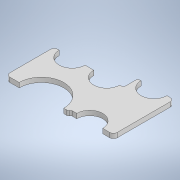
# Autodesk Inventor part: Top Bottle Middle
Saved by Autodesk Inventor 2021 (Build 250183000, 183)
## iProperties
Created: 2020-09-03
Part Number: Top Bottle Middle
Material: Generic
Document SubType Name: Modeling
Designer: jgray
Density: 1 g/cm^3
Appearance: Default
Author: jgray
Autodesk Inventor part; units mm, degrees
ref_plane "YZ Plane" through (0, 0, 0) normal (1, 0, 0) x (0, 1, 0)
ref_plane "XZ Plane" through (0, 0, 0) normal (0, 1, 0) x (-1, 0, 0)
ref_plane "XY Plane" through (0, 0, 0) normal (0, 0, 1) x (1, 0, 0)
sketch "Sketch1" plane through (0, 0, 0) normal (0, 1, 0) x (-1, 0, 0)
  circle A0 centre (18.5, 28) radius 23.85
  circle A1 centre (37, -23.25) radius 13.85
  circle A2 centre (-35, -38.75) radius 13.85
  circle A3 centre (-30.9, 25.8) radius 13.85
  circle A4 centre (0, -23.25) radius 13.85
  line L0 (56.25, 58.25) -> (-56.25, 58.25)
  line L1 (-56.25, -58.25) -> (56.25, -58.25)
  line L2 (0, -105.9299) -> (0, 123.2086) construction
  line L3 (-76.4777, -38.75) -> (-5.35, -38.75) construction
  line L4 (-123.5447, -23.25) -> (82.5572, -23.25) construction
  line L5 (56.25, -58.25) -> (56.25, 58.25)
  line L6 (56.25, 58.25) -> (56.25, -58.25)
  line L7 (-56.25, 58.25) -> (-56.25, -58.25)
  line L8 (100.0459, 28) -> (-13.85, 28) construction
  line L9 (-9.7154, 25.8) -> (-68.4996, 25.8) construction
  line L10 (18.5, 82.6038) -> (18.5, -4.654) construction
  line L11 (-30.9, 82.6038) -> (-30.9, 8.6393) construction
  point P0 (0, 0)
  point P1 (0, 0)
  dimension "d0" = 47.7
  dimension "d1" = 27.7
  dimension "d2" = 27.7
  dimension "d3" = 27.7
  dimension "d4" = 27.7
  dimension "d7" = 37
  dimension "d9" = 30.9
  dimension "d10" = 19.5
  dimension "d11" = 35
  dimension "d12" = 35
  dimension "d13" = 25.8
  dimension "d14" = 28
  dimension "d15" = 56.25
  dimension "d16" = 58.25
  dimension "d17" = 116.5
  dimension "d18" = 112.5
  dimension "d19" = 18.5
  dimension "d20" = 32.45
  constraints: 24 end point, 10 point on line, 5 centre point, 3 parallel, 2 horizontal, 2 perpendicular, 1 collinear, 1 vertical
  measures "d0" diameter of A0
  measures "d1" diameter of A1
  measures "d2" diameter of A2
  measures "d3" diameter of A3
  measures "d4" diameter of A4
  measures "d7" distance of A4.centre A1.centre
  measures "d9" distance from line of A3.centre L2
  measures "d10" distance between parallel lines of L1 L3
  measures "d11" distance between parallel lines of L1 L4
  measures "d12" horizontal distance of A2.centre A4.centre
  measures "d13" vertical distance of point (0, 0) A3.centre
  measures "d14" vertical distance of point (0, 0) A0.centre
  measures "d15" distance from line of point (0, 0) L5
  measures "d16" distance from line of L1 point (0, 0)
  measures "d17" distance between parallel lines of L1 L0
  measures "d18" distance between parallel lines of L7 L5
  measures "d19" horizontal distance of A0.centre point (0, 0)
  measures "d20" distance between parallel lines of L0 L9
extrude "Extrusion1" add sketch "Sketch1" along normal blind 5
sketch "Sketch2" plane through (0, 5, 0) normal (0, 1, 0) x (1, 0, 0)
  line L0 (-56.25, 58.25) -> (-56.25, -58.25) projected
  line L1 (-56.25, -58.25) -> (56.25, -58.25) projected
  line L2 (56.25, -58.25) -> (56.25, 58.25) projected
  line L3 (56.25, 58.25) -> (-56.25, 58.25) projected
  circle A0 centre (0, 23.25) radius 13.85 projected
  circle A1 centre (30.9, -25.8) radius 13.85 projected
  circle A2 centre (35, 38.75) radius 13.85 projected
  circle A3 centre (-37, 23.25) radius 13.85 projected
  circle A4 centre (-18.5, -28) radius 23.85 projected
  line L4 (-56.25, 58.25) -> (-56.25, -58.25) projected
  line L5 (-56.25, 23.25) -> (15.75, 23.25)
  line L6 (19.75, 38.75) -> (56.25, 38.75)
  line L7 (56.25, -58.25) -> (56.25, 58.25) projected
  line L8 (17.75, 25.25) -> (17.75, 36.75)
  arc A5 (15.75, 23.25) -> (17.75, 25.25) centre (15.75, 25.25) ccw
  arc A6 (19.75, 38.75) -> (17.75, 36.75) centre (19.75, 36.75) ccw
  point P0 (0, 0)
  point P1 (17.75, 23.25)
  point P2 (17.75, 38.75)
  point P3 (-50.85, 23.25)
  point P4 (-23.15, 23.25)
  point P5 (-13.85, 23.25)
  point P6 (13.85, 23.25)
  point P7 (21.15, 38.75)
  point P8 (48.85, 38.75)
  dimension "d23" = 74
  dimension "d25" = 38.5
  dimension "d26" = 2
  dimension "d27" = 35
  dimension "d28" = 19.5
  constraints: 6 end point, 6 point on line, 4 point on circle, 4 tangent, 2 centre point, 1 equal radius, 1 horizontal, 1 parallel, 1 vertical
  measures "d23" distance of point (17.75, 23.25) L5.start
  measures "d25" distance of point (17.75, 38.75) L6.end
  measures "d26" radius of A5
  measures "d27" distance between parallel lines of L3 L5
  measures "d28" distance between parallel lines of L3 L6
sketch "Sketch3" plane through (0, 5, 0) normal (0, 1, 0) x (1, 0, 0)
  line L0 (-56.25, -28) -> (8.75, -28)
  line L1 (12.3221, -25.8) -> (56.25, -25.8)
  line L2 (-56.25, 58.25) -> (-56.25, -58.25) projected
  line L3 (-56.25, -58.25) -> (56.25, -58.25) projected
  line L4 (56.25, -58.25) -> (56.25, 58.25) projected
  line L5 (56.25, 58.25) -> (-56.25, 58.25) projected
  circle A0 centre (0, 23.25) radius 13.85 projected
  circle A1 centre (30.9, -25.8) radius 13.85 projected
  circle A2 centre (35, 38.75) radius 13.85 projected
  circle A3 centre (-37, 23.25) radius 13.85 projected
  circle A4 centre (-18.5, -28) radius 23.85 projected
  line L6 (56.25, -58.25) -> (56.25, 58.25) projected
  line L7 (-56.25, 58.25) -> (-56.25, -58.25) projected
  line L8 (10.75, -26) -> (10.75, -25.8)
  arc A5 (8.75, -28) -> (10.5361, -26.9) centre (8.75, -26) ccw
  arc A6 (12.3221, -25.8) -> (10.5361, -26.9) centre (12.3221, -27.8) ccw
  point P0 (0, 0)
  point P1 (10.75, -28)
  point P2 (44.75, -25.8)
  point P3 (17.05, -25.8)
  point P4 (5.35, -28)
  point P5 (-42.35, -28)
  dimension "d29" = 67
  dimension "d30" = 2
  constraints: 7 point on line, 6 end point, 5 point on circle, 4 tangent, 2 centre point, 2 horizontal, 1 equal radius, 1 vertical
  measures "d29" distance of L0.start point (10.75, -28)
  measures "d30" radius of A5
extrude "Extrusion2" cut sketch "Sketch3" against normal blind 10 contours L0 A5 A6 L1 A1 L4 L3 L2 A4
extrude "Extrusion3" cut sketch "Sketch2" against normal through all contours L3 L2 L6 A2 A6 L8 A5 L5 A0 A3 L0
fillet "Fillet1" radius 4 4 edges at (-56.25, 2.5, -23.25) (-56.25, 2.5, 28) (56.25, 2.5, 25.8) (56.25, 2.5, -38.75)
body "Solid1"
